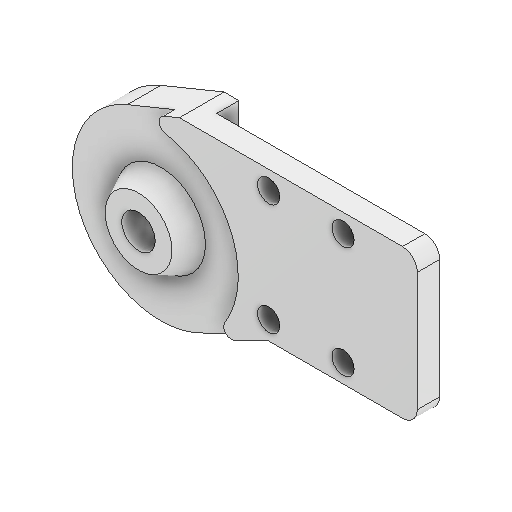
# Autodesk Inventor part: UpperCarriagePivotMount
Saved by Autodesk Inventor 2026.2 (Build 302298000, 298)
## iProperties
Created: 2026-03-25
Part Number: UpperCarriagePivotMount
Material: ABS Plastic
Document SubType Name: Modeling
Designer: gaoet
Density: 1.06 g/cm^3
Appearance: Smooth - White
Author: gaoet
Autodesk Inventor part; units mm, degrees
ref_plane "YZ Plane" through (0, 0, 0) normal (1, 0, 0) x (0, 1, 0)
ref_plane "XZ Plane" through (0, 0, 0) normal (0, 1, 0) x (-1, 0, 0)
sketch "Sketch1" plane through (0, 0, 0) normal (0, 0, 1) x (1, 0, 0)
  line L0 (-15, -10) -> (15, -10)
  line L1 (15, -10) -> (15, 10)
  line L2 (15, 10) -> (-15, 10)
  line L3 (-15, 10) -> (-15, -10)
  line L4 (-15, -10) -> (15, 10) construction
  line L5 (15, -10) -> (-15, 10) construction
  point P0 (0, 0)
  dimension "d0" = 30
  dimension "d1" = 20
  constraints: 12 end point, 2 midpoint, 2 parallel, 1 horizontal, 1 perpendicular
  measures "d0" distance of L2.end L1.end
  measures "d1" distance of L1.end L0.end
extrude "Extrusion1" add sketch "Sketch1" along normal blind 3
sketch "Sketch2" plane through (0, 0, 3) normal (0, 0, 1) x (1, 0, 0)
  line L0 (-5, -7.5) -> (5, -7.5)
  line L1 (5, -7.5) -> (5, 7.5)
  line L2 (5, 7.5) -> (-5, 7.5)
  line L3 (-5, 7.5) -> (-5, -7.5)
  line L4 (-5, -7.5) -> (5, 7.5) construction
  line L5 (5, -7.5) -> (-5, 7.5) construction
  point P0 (0, 0)
  point P1 (0, 0)
  dimension "d4" = 10
  dimension "d5" = 15
  constraints: 12 end point, 2 midpoint, 2 parallel, 1 coincident, 1 horizontal, 1 perpendicular
  measures "d4" distance of L2.end L1.end
  measures "d5" distance of L1.end L0.end
hole "Hole1" at (-5, 7.5, 3) at (5, 7.5, 3) at (-5, -7.5, 3) at (5, -7.5, 3) direction (0, 0, -1) diameter 3 end through all
sketch "Sketch3" plane through (0, 0, 3) normal (0, 0, 1) x (1, 0, 0)
  line L0 (-18.979274, -1) -> (-16.958548, -4.5)
  line L1 (-16.958548, -4.5) -> (-18.979274, -8)
  line L2 (-18.979274, -8) -> (-23.020726, -8)
  line L3 (-23.020726, -8) -> (-25.041452, -4.5)
  line L4 (-25.041452, -4.5) -> (-23.020726, -1)
  line L5 (-23.020726, -1) -> (-18.979274, -1)
  circle A0 centre (-21, -4.5) radius 11.90625
  line L6 (15, -10) -> (15, 10)
  line L7 (15, 10) -> (-15, 10)
  line L8 (-15, 10) -> (-15, -10)
  line L9 (-15, -10) -> (15, -10)
  line L10 (-100, -4.5) -> (100, -4.5) construction
  line L11 (100, -4.5) -> (100, 4.5) construction
  line L12 (100, 4.5) -> (-100, 4.5) construction
  line L13 (-100, 4.5) -> (-100, -4.5) construction
  line L14 (-100, -4.5) -> (100, 4.5) construction
  line L15 (100, -4.5) -> (-100, 4.5) construction
  line L16 (-15, 10) -> (-17, 10)
  line L17 (-17, 10) -> (-25.507677, 6.519965)
  line L18 (15, -10) -> (15, -12)
  line L19 (15, -12) -> (-19.52358, -16.314354)
  line L20 (-22.587713, -1.75) -> (-19.412287, -1.75) construction
  line L21 (-19.412287, -1.75) -> (-17.824574, -4.5) construction
  line L22 (-17.824574, -4.5) -> (-19.412287, -7.25) construction
  line L23 (-19.412287, -7.25) -> (-22.587713, -7.25) construction
  line L24 (-22.587713, -7.25) -> (-24.175426, -4.5) construction
  line L25 (-24.175426, -4.5) -> (-22.587713, -1.75) construction
  circle A1 centre (-21, -4.5) radius 2 construction
  circle A2 centre (-21, -4.5) radius 1.5 construction
  line L26 (-5, -10) -> (-15.826239, -15.223385)
  point P0 (0, 0)
  point P1 (-21, -1)
  point P2 (-17.377304, -15.841731)
  point P3 (-10.440228, -10)
  point P4 (-15, 5.783909)
  point P5 (15, -11)
  dimension "d13" = 7
  dimension "d14" = 23.8125
  dimension "d15" = 9
  dimension "d16" = 200
  dimension "d19" = 4.5
  dimension "d30" = 21
  dimension "d44" = 2
  dimension "d46" = 5.5
  dimension "d47" = 4
  dimension "d48" = 0
  dimension "d49" = 3
  dimension "d73" = 20
  constraints: 46 end point, 4 coincident, 4 horizontal, 4 midpoint, 4 point on circle, 3 centre point, 3 tangent, 2 parallel, 2 perpendicular, 1 point on line, 1 vertical, 26 other
  measures "d13" distance from line of L2 point (-21, -1)
  measures "d14" diameter of A0
  measures "d15" distance of L11.end L10.end
  measures "d16" distance of L11.end L12.end
  measures "d19" vertical distance of point (0, 0) point (-21, -4.5)
  measures "d30" horizontal distance of point (0, 0) point (-21, -4.5)
  measures "d44" distance of L7.end L16.end
  measures "d46" distance between parallel lines of L23 L20
  measures "d47" diameter of A1
  measures "d48" distance from line of L10 point (-21, -4.5)
  measures "d49" diameter of A2
  measures "d73" horizontal distance of point (15, -11) L26.start
extrude "Extrusion2" add sketch "Sketch3" against normal up to surface (3 mm away) contours L0 L1 L2 L3 L4 L5 | A0 L8 L9 | L17 L16 L8 A0 | A0 L9 L8 | A0 L9 L26
sketch "Sketch4" plane through (0, 0, 0) normal (0, 0, -1) x (-1, 0, 0)
  line L0 (-15, -10) -> (-15, 10)
  arc A0 (15.826239, -15.223385) -> (25.507677, 6.519965) centre (21, -4.5) ccw
  line L1 (-15, 10) -> (17, 10)
  line L2 (15, -10) -> (-15, -10)
  line L3 (-15, -10) -> (-15, 10)
  line L4 (-15, 10) -> (15, 10)
  line L5 (15, 10) -> (15, -10)
  line L6 (15, -10) -> (-15, 10) construction
  line L7 (-15, -10) -> (15, 10) construction
  line L8 (25.507677, 6.519965) -> (17, 10)
  line L9 (5, -10) -> (15.826239, -15.223385)
  line L10 (5, -10) -> (-15, -10)
  point P0 (0, 0)
  point P1 (15, 1.283909)
  point P2 (9.135819, -10)
  constraints: 12 end point, 2 midpoint, 2 parallel, 1 horizontal, 1 perpendicular
extrude "Extrusion3" add sketch "Sketch4" along normal blind 3 contours L2 L5 L1 L8 A0 L9
sketch "Sketch5" plane through (0, 0, -3) normal (0, 0, -1) x (-1, 0, 0)
  arc A0 (15.826239, -15.223385) -> (25.507677, 6.519965) centre (21, -4.5) ccw
  line L0 (15, -10) -> (5, -10)
  line L1 (15, -5) -> (32.895747, -5)
  line L2 (100, -4.5) -> (-100, -4.5) construction
  line L3 (17, 10) -> (15, 10)
  line L4 (25.507677, 6.519965) -> (17, 10)
  line L5 (5, -10) -> (15.826239, -15.223385)
  line L6 (15, 10) -> (15, -10)
  point P0 (0, 0)
  dimension "d25" = 0.5
  constraints: 2 end point, 1 horizontal, 1 point on circle
  measures "d25" distance between parallel lines of L1 L2
extrude "Extrusion4" add sketch "Sketch5" along normal blind 6
extrude "Extrusion5" cut sketch "Sketch3" against normal blind 1.5 contours L0 L1 L2 L3 L4 L5 | A0 L8 L9 | A0 L9 L8
fillet "Fillet1" radius 1 2 edges at (-25.5077, 6.52, 2.25) (-15.8262, -15.2234, 2.25)
sketch "Sketch6" plane through (0, 0, 1.5) normal (0, 0, 1) x (1, 0, 0)
  arc A0 (-25.507677, 6.519965) -> (-15.826239, -15.223385) centre (-21, -4.5) ccw
  arc A1 (-10.894095, -10.795194) -> (-18.916677, 7.222566) centre (-21, -4.5) ccw
  arc A2 (-19.120298, 9.1327) -> (-18.916677, 7.222566) centre (-18.7417, 8.207139) ccw
  line L0 (-19.120298, 9.1327) -> (-25.507677, 6.519965)
  line L1 (-15.826239, -15.223385) -> (-9.610763, -12.224576)
  arc A3 (-10.894095, -10.795194) -> (-9.610763, -12.224576) centre (-10.045305, -11.323924) ccw
  point P0 (0, 0)
hole "Hole2" at (-21, -4.5, 1.5) direction (0, 0, -1) diameter 4.5 depth 4
sketch "Sketch7" plane through (0, 0, -9) normal (0, 0, -1) x (-1, 0, 0)
  arc A0 (15.826239, -15.223385) -> (25.507677, 6.519965) centre (21, -4.5) ccw
  line L0 (15, -10) -> (5, -10)
  line L1 (18.979274, -1) -> (23.020726, -1)
  line L2 (23.020726, -1) -> (25.041452, -4.5)
  line L3 (25.041452, -4.5) -> (23.020726, -8)
  line L4 (23.020726, -8) -> (18.979274, -8)
  line L5 (18.979274, -8) -> (16.958548, -4.5)
  line L6 (16.958548, -4.5) -> (18.979274, -1)
  line L7 (25.507677, 6.519965) -> (17, 10)
  line L8 (17, 10) -> (15, 10)
  line L9 (5, -10) -> (15.826239, -15.223385)
  line L10 (15, 10) -> (15, -10)
  point P0 (0, 0)
  point P1 (21, -8)
  dimension "d39" = 7
  constraints: 12 end point, 1 coincident, 1 horizontal, 1 midpoint, 13 other
  measures "d39" distance from line of point (21, -8) L1
extrude "Extrusion6" cut sketch "Sketch7" against normal blind 4 contours L9 L0 L10 L8 L7 A0 | L1 L2 L3 L4 L5 L6
sketch "Sketch9" plane through (0, 0, -5) normal (0, 0, -1) x (-1, 0, 0)
  arc A0 (15.826239, -15.223385) -> (25.507677, 6.519965) centre (21, -4.5) ccw
  circle A1 centre (21, -7) radius 6
  line L0 (27, -7) -> (27, -5)
  line L1 (15, -7) -> (15, -5)
  line L2 (15, -10) -> (15.803848, -10)
  line L3 (15, 10) -> (17, 10)
  line L4 (15.826239, -15.223385) -> (5, -10)
  line L5 (17, 10) -> (25.507677, 6.519965)
  line L6 (15, -10) -> (15, 10)
  line L7 (5, -10) -> (15, -10)
  point P0 (0, 0)
  dimension "d52" = 12
  constraints: 6 end point, 3 point on circle, 2 tangent, 1 centre point, 1 horizontal, 1 parallel, 1 vertical
  measures "d52" diameter of A1
extrude "Extrusion8" [suppressed]
chamfer "Chamfer1" [suppressed]
sketch "Sketch11" plane through (0, 0, 1.5) normal (0, 0, 1) x (1, 0, 0)
  circle A0 centre (-21, -4.5) radius 2.25
  arc A1 (-25.507677, 6.519965) -> (-15.826239, -15.223385) centre (-21, -4.5) ccw
  arc A2 (-10.894095, -10.795194) -> (-18.916677, 7.222566) centre (-21, -4.5) ccw
  arc A3 (-19.120298, 9.1327) -> (-18.916677, 7.222566) centre (-18.7417, 8.207139) ccw
  line L0 (-19.120298, 9.1327) -> (-25.507677, 6.519965)
  circle A4 centre (-21, -4.5) radius 4.5
  line L1 (-15.826239, -15.223385) -> (-9.610763, -12.224576)
  arc A5 (-10.894095, -10.795194) -> (-9.610763, -12.224576) centre (-10.045305, -11.323924) ccw
  point P0 (0, 0)
  dimension "d61" = 9
  constraints: 1 centre point, 1 coincident
  measures "d61" diameter of A4
extrude "Extrusion10" add sketch "Sketch11" along normal blind 3 contours A4
chamfer "Chamfer2" distance 1.5 distance2 3 1 edges at (-25.5, -4.5, 1.5) measured on face at (-15.1038, -11.5542, 1.5)
sketch "Sketch12" plane through (0, 0, -5) normal (0, 0, -1) x (-1, 0, 0)
  circle A0 centre (21, -4.5) radius 4.5
  line L0 (23.020726, -8) -> (18.979274, -8)
  line L1 (18.979274, -8) -> (16.958548, -4.5)
  line L2 (16.958548, -4.5) -> (18.979274, -1)
  line L3 (18.979274, -1) -> (23.020726, -1)
  line L4 (23.020726, -1) -> (25.041452, -4.5)
  line L5 (25.041452, -4.5) -> (23.020726, -8)
  point P0 (0, 0)
  point P1 (21, -8)
  dimension "d67" = 7
  constraints: 12 end point, 1 coincident, 1 horizontal, 1 midpoint, 13 other
  measures "d67" distance from line of point (21, -8) L3
extrude "Extrusion11" cut sketch "Sketch12" against normal blind 5.5 contours L0 L1 L2 L3 L4 L5
sketch "Sketch13" plane through (0, 0, -5) normal (0, 0, -1) x (-1, 0, 0)
  line L0 (25.041452, -4.5) -> (23.020726, -8)
  line L1 (23.020726, -8) -> (18.979274, -8)
  line L2 (18.979274, -8) -> (16.958548, -4.5)
  arc A0 (15.826239, -15.223385) -> (25.507677, 6.519965) centre (21, -4.5) ccw
  line L3 (25.041452, -7) -> (25.041452, -5)
  line L4 (16.958548, -7) -> (16.958548, -5)
  line L5 (18.979274, -1) -> (23.020726, -1)
  line L6 (23.020726, -1) -> (25.041452, -4.5)
  line L7 (16.958548, -4.5) -> (18.979274, -1)
  line L8 (15, 10) -> (17, 10)
  line L9 (15.826239, -15.223385) -> (5, -10)
  line L10 (17, 10) -> (25.507677, 6.519965)
  line L11 (15, -10) -> (15, 10)
  line L12 (5, -10) -> (15, -10)
  point P0 (0, 0)
  constraints: 4 end point, 2 vertical
extrude "Extrusion12" cut sketch "Sketch13" against normal up to surface (2 mm away)
ref_plane "Work Plane1" through (0, 0, 1.35) normal (0, 0, 1) x (1, 0, 0)
fillet "Fillet4" radius 2 2 edges at (15, -10, 1.5) (15, 10, 1.5)
body "Solid1"
